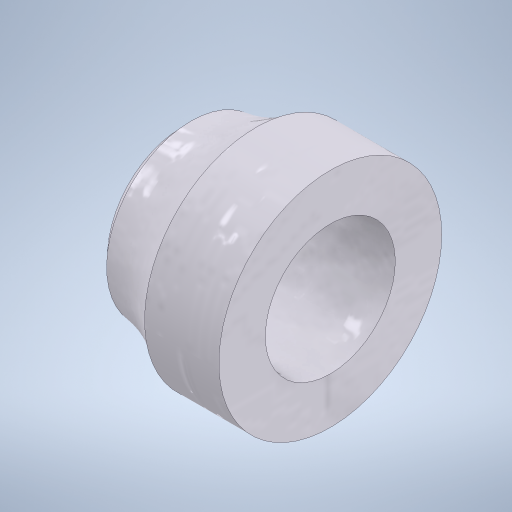
# Autodesk Inventor part: Cover
Saved by Autodesk Inventor 2024 (Build 280153000, 153)
## iProperties
Created: 2024-03-07
Part Number: Cover
Material: Aluminum 6061, geschweißt
Document SubType Name: Modeling
Designer: ffogue
Density: 2.7 g/cm^3
Appearance: Schweißnaht - Aluminum
Author: ffogue
Autodesk Inventor part; units mm, degrees
ref_plane "YZ Plane" through (0, 0, 0) normal (1, 0, 0) x (0, 1, 0)
ref_plane "XZ Plane" through (0, 0, 0) normal (0, 1, 0) x (-1, 0, 0)
ref_plane "XY Plane" through (0, 0, 0) normal (0, 0, 1) x (1, 0, 0)
sketch "Skizze1" plane through (0, 0, 0) normal (0, 0, 1) x (1, 0, 0)
  line L0 (0, 0) -> (8, 0)
  line L1 (0, 0) -> (0, 4.5)
  line L2 (0, 4.5) -> (4, 4.5)
  line L3 (4, 4.5) -> (4, 6)
  line L4 (4, 6) -> (8, 6)
  line L5 (8, 6) -> (8, 0)
  dimension "d0" = 8
  dimension "d1" = 12
  dimension "d2" = 9
  dimension "d3" = 4
  constraints: 12 end point, 4 perpendicular, 1 coincident, 1 horizontal, 1 vertical
  measures "d0" distance of L0.start L0.end
  measures "d1" diameter of L4 L0
  measures "d2" diameter of L2 L0
  measures "d3" distance between parallel lines of L3 L1
revolve "Umdrehung1" add sketch "Skizze1" angle 360 about axis through (0, 0, 0) along (1, 0, 0)
fillet "Rundung1" radius 7 1 edges at (4, -4.5, 0)
sketch "Skizze2" plane through (0, 0, 0) normal (-1, 0, 0) x (0, 0, 1)
  circle A0 centre (0, 0) radius 4.5 projected
  constraints: 1 coincident
hole "Bohrung1" at (0, 0, 0) direction (1, 0, 0) diameter 7 end through all
chamfer "Fasen1" distance 0.5 angle 45 1 edges at (0, -4.5, 0)
